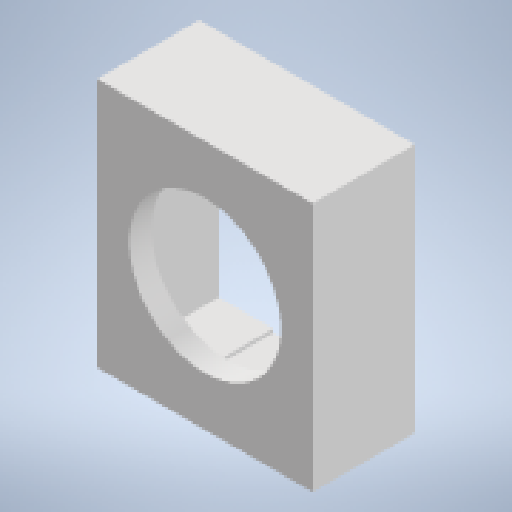
# Autodesk Inventor part: bau_holder
Saved by Autodesk Inventor 2024.2 (Build 282272000, 272)
## iProperties
Created: 2023-11-11
Part Number: bau_holder
Material: Generic
Document SubType Name: Modeling
Designer: adrie
Density: 1 g/cm^3
Appearance: Default
Author: adrie
Autodesk Inventor part; units mm, degrees
ref_plane "YZ Plane" through (0, 0, 0) normal (1, 0, 0) x (0, 1, 0)
ref_plane "XZ Plane" through (0, 0, 0) normal (0, 1, 0) x (-1, 0, 0)
sketch "Sketch1" plane through (0, 0, 0) normal (0, 0, 1) x (1, 0, 0)
  line L0 (-11, 18.9) -> (-11, 18.25) projected
  line L1 (-11, 18.25) -> (-20.7, 18.25) projected
  line L2 (-20.7, 18.25) -> (-20.7, -18.25) projected
  line L3 (-11, -18.25) -> (-20.7, -18.25) projected
  line L4 (-11, -18.25) -> (-11, -18.9) projected
  line L5 (0, -18.9) -> (-11, -18.9) projected
  line L6 (0, -18.25) -> (0, -18.9) projected
  line L7 (9.7, -18.25) -> (0, -18.25) projected
  line L8 (9.7, 18.25) -> (9.7, -18.25) projected
  line L9 (9.7, 18.25) -> (0, 18.25) projected
  line L10 (0, 18.9) -> (0, 18.25) projected
  line L11 (0, 18.9) -> (-11, 18.9) projected
  circle A0 centre (-5.5, 0) radius 11.5 projected
  circle A1 centre (-5.5, 0) radius 13.5
  point P0 (0, 0)
  dimension "d0" = 2
  constraints: 1 centre point, 1 coincident
  measures "d0" radial gap between concentric circles of A0 A1
extrude "Extrusion1" add sketch "Sketch1" along normal blind 4 contours L11 L10 L9 L8 L7 L6 L5 L4 L3 L2 L1 L0
sketch "Sketch2" plane through (0, 0, 4) normal (0, 0, 1) x (1, 0, 0)
  line L0 (-11, 18.9) -> (-11, 18.25) projected
  line L1 (-11, 18.25) -> (-20.7, 18.25) projected
  line L2 (-20.7, 18.25) -> (-20.7, -18.25) projected
  line L3 (-20.7, -18.25) -> (-11, -18.25) projected
  line L4 (-11, -18.25) -> (-11, -18.9) projected
  line L5 (-11, -18.9) -> (0, -18.9) projected
  line L6 (0, -18.9) -> (0, -18.25) projected
  line L7 (0, -18.25) -> (9.7, -18.25) projected
  line L8 (9.7, -18.25) -> (9.7, 18.25) projected
  line L9 (9.7, 18.25) -> (0, 18.25) projected
  line L10 (0, 18.25) -> (0, 18.9) projected
  line L11 (0, 18.9) -> (-11, 18.9) projected
  circle A0 centre (-5.5, 0) radius 13.5 projected
  line L12 (13.7, 22.25) -> (13.7, -22.25)
  line L13 (13.7, -22.25) -> (6, -22.25)
  line L14 (-17, -22.25) -> (-24.7, -22.25)
  line L15 (-24.7, -22.25) -> (-24.7, 22.25)
  line L16 (-24.7, 22.25) -> (-17, 22.25)
  line L17 (6, 22.25) -> (13.7, 22.25)
  line L18 (10.2, 18.75) -> (10.2, -18.75)
  line L19 (10.2, -18.75) -> (0.5, -18.75)
  line L20 (0.5, -18.75) -> (0.5, -19.4)
  line L21 (0.5, -19.4) -> (-11.5, -19.4)
  line L22 (-11.5, -19.4) -> (-11.5, -18.75)
  line L23 (-11.5, -18.75) -> (-21.2, -18.75)
  line L24 (-21.2, -18.75) -> (-21.2, 18.75)
  line L25 (-21.2, 18.75) -> (-11.5, 18.75)
  line L26 (-11.5, 18.75) -> (-11.5, 19.4)
  line L27 (-11.5, 19.4) -> (0.5, 19.4)
  line L28 (0.5, 19.4) -> (0.5, 18.75)
  line L29 (0.5, 18.75) -> (10.2, 18.75)
  line L30 (-17, -22.25) -> (6, -22.25)
  line L31 (6, 22.25) -> (-17, 22.25)
  point P0 (0, 0)
  dimension "d3" = 4
  dimension "d4" = 0.5
  constraints: 40 end point, 1 collinear, 1 horizontal, 14 other
  measures "d3" distance between parallel lines of L8 L12
  measures "d4" distance between parallel lines of L8 L18
ref_plane "Work Plane1" through (-21.9731, -18.5883, -14.2) normal (0, 0, -1) x (0, 1, 0)
extrude "Extrusion2" add sketch "Sketch2" against normal up to surface (18.2 mm away) contours L12 L13 L30 L14 L15 L16 L31 L17
extrude "Extrusion3" add sketch "Sketch2" against normal blind 4 contours L18 L19 L20 L21 L22 L23 L24 L25 L26 L27 L28 L29
sketch "Sketch3" plane through (-24.7, -22.25, 4) normal (-1, 0, 0) x (0, 0, 1)
  line L0 (0, 44.5) -> (-18.2, 44.5) construction
  line L1 (-18.2, 44.5) -> (0, 0) construction
  line L2 (0, 0) -> (-18.2, 0) construction
  line L3 (0, 44.5) -> (0, 0) construction
  line L4 (-18.2, 0) -> (0, 44.5) construction
  line L5 (0, 44.5) -> (-9.1, 22.25) construction
  line L6 (0, 22.25) -> (-18.2, 22.25) construction
  line L7 (-18.2, 3.5) -> (-18.2, 41) construction
  line L8 (-18.2, 22.25) -> (0, 44.5) construction
  line L9 (0, 22.25) -> (-18.2, 44.5) construction
  line L10 (-9.1, 33.375) -> (0, 33.375) construction
  line L11 (0, 33.375) -> (-18.2, 44.5) construction
  line L12 (0, 44.5) -> (-18.2, 33.375) construction
  line L13 (-18.2, 44.5) -> (-18.2, 0) construction
  circle A0 centre (-9.1, 38.9375) radius 1.6
  circle A1 centre (-9.1, 5.5625) radius 1.6
  point P0 (-4, 22.25)
  dimension "d9" = 3.2
  constraints: 20 end point, 5 midpoint, 2 centre point, 2 point on line, 1 parallel, 1 perpendicular, 1 symmetric about line, 1 other
  measures "d9" diameter of A0
extrude "Extrusion4" cut sketch "Sketch3" against normal through all
sketch "Sketch4" plane through (-24.7, 22.25, 4) normal (0, 1, 0) x (1, 0, 0)
  line L0 (0, 0) -> (0, 18.2) construction
  line L1 (38.4, 18.2) -> (0, 0) construction
  line L2 (0, 0) -> (0, 18.2) construction
  line L3 (0, 18.2) -> (38.4, 0) construction
  circle A0 centre (19.2, 9.1) radius 1.6
  point P0 (24.7, 4)
  dimension "d12" = 3.2
  constraints: 6 end point, 1 centre point, 1 collinear, 1 midpoint
  measures "d12" diameter of A0
extrude "Extrusion5" cut sketch "Sketch4" against normal through all
sketch "Sketch5" plane through (0, 0, 4) normal (0, 0, 1) x (1, 0, 0)
  line L0 (13.7, 22.25) -> (-24.7, 22.25) projected
  line L1 (13.7, 22.25) -> (-24.7, 22.25)
  line L2 (-24.7, 22.25) -> (-24.7, 32.25)
  line L3 (-24.7, 32.25) -> (13.7, 32.25)
  line L4 (13.7, 32.25) -> (13.7, 22.25)
  line L5 (-24.7, 22.25) -> (-24.7, -22.25) projected
  line L6 (-24.7, 22.25) -> (-34.7, 22.25)
  line L7 (-34.7, 22.25) -> (-34.7, -22.25)
  line L8 (-34.7, -22.25) -> (-24.7, -22.25)
  line L9 (-24.7, -22.25) -> (-24.7, 22.25)
  line L10 (13.7, 27.25) -> (-24.7, 27.25) construction
  line L11 (-29.7, 22.25) -> (-29.7, -22.25) construction
  circle A0 centre (8.7, 27.25) radius 1.6
  circle A1 centre (-29.7, -17.25) radius 1.6
  circle A2 centre (-29.7, -7.25) radius 1.6
  line L12 (-24.7, 0) -> (-34.7, 0) construction
  circle A3 centre (-29.7, 17.25) radius 1.6
  circle A4 centre (-29.7, 7.25) radius 1.6
  line L13 (-5.5, 22.25) -> (-5.5, 32.25) construction
  circle A5 centre (-1.3, 27.25) radius 1.6652
  circle A6 centre (-19.7, 27.25) radius 1.6
  circle A7 centre (-9.7, 27.25) radius 1.6652
  line L14 (13.7, 22.25) -> (-24.7, 22.25) projected
  line L15 (-24.7, 22.25) -> (-24.7, -22.25) projected
  line L16 (-24.7, -22.25) -> (13.7, -22.25) projected
  line L17 (13.7, -22.25) -> (13.7, 22.25) projected
  circle A8 centre (-5.5, 0) radius 13.5 projected
  point P0 (0, 0)
  dimension "d15" = 10
  dimension "d16" = 10
  dimension "d17" = 3.2
  dimension "d18" = 5
  dimension "d19" = 3.2
  dimension "d20" = 5
  dimension "d21" = 10
  dimension "d22" = 3.2
  dimension "d23" = 10
  constraints: 24 end point, 8 centre point, 8 midpoint, 4 parallel, 4 point on line, 4 symmetric about line, 2 horizontal, 2 perpendicular, 4 other
  measures "d15" distance of L3.end L0.start
  measures "d16" distance of L7.end L8.end
  measures "d17" diameter of A0
  measures "d18" distance from line of L4 A0.centre
  measures "d19" diameter of A1
  measures "d20" distance from line of L8 A1.centre
  measures "d21" distance of A1.centre A2.centre
  measures "d22" diameter of A2
  measures "d23" distance of A0.centre A5.centre
extrude "Extrusion6" add sketch "Sketch5" along normal blind 2.5
body "Solid1"
